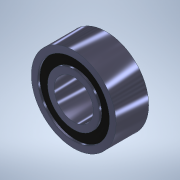
# Autodesk Inventor part: 6202-2rs_15x35x11
Saved by Autodesk Inventor 2022 (Build 260153000, 153)
## iProperties
Created: 2016-09-14
Part Number: 6202-2rs_15x35x11
Material: Steel
Document SubType Name: Modeling
Designer: Kostic
Density: 7.85 g/cm^3
Appearance: Steel Blue
Mass: 4.21712 g
Surface Area: 7.16283 cm^2
Volume: 0.537212 cm^3
Author: Kostic
Autodesk Inventor part; units mm, degrees
ref_plane "YZ Plane" through (0, 0, 0) normal (1, 0, 0) x (0, 1, 0)
ref_plane "XZ Plane" through (0, 0, 0) normal (0, 1, 0) x (-1, 0, 0)
ref_plane "XY Plane" through (0, 0, 0) normal (0, 0, 1) x (1, 0, 0)
sketch "Sketch1" plane through (0, 0, 0) normal (0, 0, 1) x (1, 0, 0)
  line L0 (0, 0) -> (0, 10) construction
  line L1 (0, 0) -> (10, 0) construction
  line L2 (3, 2.5) -> (4, 2.5)
  line L3 (4, 2.5) -> (4, -2.5)
  line L4 (4, -2.5) -> (3, -2.5)
  line L5 (3, -2.5) -> (3, 2.5)
  line L6 (4, 2.2) -> (5.5, 2.2)
  line L7 (5.5, 2.2) -> (5.5, -2.2)
  line L8 (5.5, -2.2) -> (4, -2.2)
  line L9 (4, -2.2) -> (4, 2.2)
  line L10 (5.5, 2.5) -> (6.5, 2.5)
  line L11 (6.5, 2.5) -> (6.5, -2.5)
  line L12 (6.5, -2.5) -> (5.5, -2.5)
  line L13 (5.5, -2.5) -> (5.5, 2.5)
  dimension "d0" = 10
  dimension "d1" = 90
  dimension "d2" = 1
  dimension "d3" = 5
  dimension "d5" = 4.4
  dimension "d6" = 0.3
  dimension "d7" = 2.5
  dimension "d8" = 1
  dimension "d9" = 5
  dimension "d10" = 3
  dimension "d11" = 2.5
  dimension "d13" = 6.5
  constraints: 28 end point, 6 parallel, 4 horizontal, 4 perpendicular, 1 collinear, 1 point on line, 1 vertical
  measures "d0" distance of L0.start L0.end
  measures "d1" angle of L1 L0
  measures "d2" distance of L3.end L4.end
  measures "d3" distance of L2.end L3.end
  measures "d5" distance of L6.end L7.end
  measures "d6" distance between parallel lines of L2 L6
  measures "d7" distance from line of L0.start L2
  measures "d8" distance of L11.end L12.end
  measures "d9" distance of L10.end L11.end
  measures "d10" distance from line of L0.start L5
  measures "d11" distance from line of L0.start L10
  measures "d13" distance from line of L0.start L11
revolve "Revolution1" add sketch "Sketch1" angle 360 about axis through (0, 0, 0) along (0, 1, 0)
equation "\"d5\" = d9 - 2 * d6"
equation "\"d7\" = 0.5 * d3"
equation "\"d8\" = d2"
equation "\"d9\" = d3"
equation "\"d11\" = d7"
body "Solid1"
